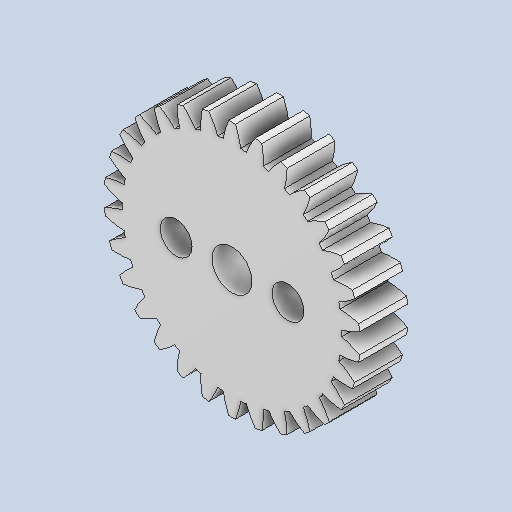
# Autodesk Inventor part: 平歯車1
Saved by Autodesk Inventor 2025.2 (Build 292293000, 293)
## iProperties
CustomPartVersion: 1
Created: 2024-12-16
Part Number: 平歯車1
Material: ABS プラスチック
Document SubType Name: Modeling
Designer: haruy
Categories: <?xml version="1.0" encoding="UTF-16"?> <MemberInstance><Categories><FamilyTemplate><FamilyTemplateParameter ValueType="xs:double" Id="1" ObjectReferenceKey="da_z" ObjectType="kUserParameterObject"/><FamilyTemplateParameter ValueType="xs:double" Id="2" ObjectReferenceKey="da_b" ObjectType="kUserParameterObject"/><FamilyTemplateParameter ValueType="xs:double" Id="3" ObjectReferenceKey="da_beta" ObjectType="kUserParameterObject"/><FamilyTemplateParameter ValueType="xs:double" Id="4" ObjectReferenceKey="da_da" ObjectType="kUserParameterObject"/><FamilyTemplateParameter ValueType="xs:double" Id="5" ObjectReferenceKey="da_aw" ObjectType="kUserParameterObject"/><FamilyTemplateParameter ValueType="xs:string" Id="6" ObjectReferenceKey="EAIAABAAAACIAQAAAAAAAIAAAAAAAAAA" ObjectType="83910656" SubObjectId="SurfaceGeometry"/></FamilyTemplate><ParamToTemplateMap><ParamToTemplate CategoryParameter="//CategoryParameter[@InternalName='046C89C9-8512-4d59-83FE-43B91F4F132A']" TemplateParameter="1"/><ParamToTemplate CategoryParameter="//CategoryParameter[@InternalName='2552DF32-E462-4b46-AEBF-C6C7768E72AC']" TemplateParameter="2"/><ParamToTemplate CategoryParameter="//CategoryParameter[@InternalName='C9EE641D-15FC-4fae-A226-E94C4372FDD7']" TemplateParameter="3"/><ParamToTemplate><ParamToTemplate CategoryParameter="//CategoryParameter[@InternalName='00B6519A-459B-49c7-AD84-2E56D39A5744']" ConstantValue="0.000000"/></ParamToTemplate><ParamToTemplate><ParamToTemplate CategoryParameter="//CategoryParameter[@InternalName='04B31F0E-C7A6-4894-AA32-9629BEFACF47']" ConstantValue="1.000000"/></ParamToTemplate><ParamToTemplate><ParamToTemplate CategoryParameter="//CategoryParameter[@InternalName='43CBEC2E-7847-49e7-A936-2F7889FCB2D9']" ConstantValue="0.250000"/></ParamToTemplate><ParamToTemplate><ParamToTemplate CategoryParameter="//CategoryParameter[@InternalName='B1EFC894-105D-4ebd-86BF-FA20ED196853']" ConstantValue="0.350000"/></ParamToTemplate><ParamToTemplate><ParamToTemplate CategoryParameter="//CategoryParameter[@InternalName='51175063-3D10-4879-93E8-6246FE8B403D']" ConstantValue="2060000000.000000"/></ParamToTemplate><ParamToTemplate><ParamToTemplate CategoryParameter="//CategoryParameter[@InternalName='A3A52E27-4454-46a9-B0BD-C932399B70AF']" ConstantValue="0.300000"/></ParamToTemplate><ParamToTemplate><ParamToTemplate CategoryParameter="//CategoryParameter[@InternalName='91B76062-C214-41d9-B1B9-14D2AB99603D']" ConstantValue="0.100000"/></ParamToTemplate><ParamToTemplate><ParamToTemplate CategoryParameter="//CategoryParameter[@InternalName='374E806E-8B8A-4dda-A9AA-1039D6500AD2']" ConstantValue="10.000000"/></ParamToTemplate><ParamToTemplate><ParamToTemplate CategoryParameter="//CategoryParameter[@InternalName='2D373A89-B862-43d6-8D0B-0CBF12AB9F6C']" ConstantValue="0.349066"/></ParamToTemplate><ParamToTemplate CategoryParameter="//CategoryParameter[@InternalName='37777632-D6A2-4fac-9D53-DB8ACD95C989']" TemplateParameter="4"/><ParamToTemplate CategoryParameter="//CategoryParameter[@InternalName='FD1017F1-B727-4f7e-9707-0F86F1FF9423']" TemplateParameter="5"/><ParamToTemplate><ParamToTemplate CategoryParameter="//CategoryParameter[@InternalName='9E1B4470-B2D3-4ff1-B813-535BB4CDF51A']" ConstantValue="3520000.000000"/></ParamToTemplate><ParamToTemplate><ParamToTemplate CategoryParameter="//CategoryParameter[@InternalName='F8452263-BFF6-458c-9FB1-07C4B99E95CD']" ConstantValue="11400000.000000"/></ParamToTemplate><ParamToTemplate><ParamToTemplate CategoryParameter="//CategoryParameter[@InternalName='3E3BB259-FD49-497f-8171-6EBC954A3479']" ConstantValue="2.000000"/></ParamToTemplate><ParamToTemplate CategoryParameter="//CategoryParameter[@InternalName='27C3BAF2-7550-4e4b-AE2C-0DB134B7D9B7']" TemplateParameter="6"/></ParamToTemplateMap><Category DisplayName="Gear" InternalName="DC85795E-93AB-48d5-8EEE-5A27447B64BD" Mnemonic="Gear"><CategoryParameter DisplayName="z" InternalName="046C89C9-8512-4d59-83FE-43B91F4F132A" Mnemonic="z"/><CategoryParameter DisplayName="b" InternalName="2552DF32-E462-4b46-AEBF-C6C7768E72AC" Mnemonic="b"/><CategoryParameter DisplayName="||b|" InternalName="C9EE641D-15FC-4fae-A226-E94C4372FDD7" Mnemonic="beta"/><CategoryParameter DisplayName="x" InternalName="00B6519A-459B-49c7-AD84-2E56D39A5744" Mnemonic="x"/><CategoryParameter DisplayName="a*" InternalName="04B31F0E-C7A6-4894-AA32-9629BEFACF47" Mnemonic="a"/><CategoryParameter DisplayName="c*" InternalName="43CBEC2E-7847-49e7-A936-2F7889FCB2D9" Mnemonic="c"/><CategoryParameter DisplayName="r|.f|*" InternalName="B1EFC894-105D-4ebd-86BF-FA20ED196853" Mnemonic="rf"/><CategoryParameter DisplayName="E" InternalName="51175063-3D10-4879-93E8-6246FE8B403D" Mnemonic="E"/><CategoryParameter DisplayName="||m|" InternalName="A3A52E27-4454-46a9-B0BD-C932399B70AF" Mnemonic="mi"/><Category DisplayName="SpurGear" InternalName="26C5A22E-A91E-4dfd-A3B3-23CCAFAE1764" Mnemonic="SpurGear"><CategoryParameter DisplayName="m" InternalName="91B76062-C214-41d9-B1B9-14D2AB99603D" Mnemonic="m"/><CategoryParameter DisplayName="P" InternalName="374E806E-8B8A-4dda-A9AA-1039D6500AD2" Mnemonic="PP"/><CategoryParameter DisplayName="||a|" InternalName="2D373A89-B862-43d6-8D0B-0CBF12AB9F6C" Mnemonic="alpha"/><CategoryParameter DisplayName="d|.a|" InternalName="37777632-D6A2-4fac-9D53-DB8ACD95C989" Mnemonic="da"/><CategoryParameter DisplayName="a|.w|" InternalName="FD1017F1-B727-4f7e-9707-0F86F1FF9423" Mnemonic="aw"/><CategoryParameter DisplayName="||s||.Flim|" InternalName="9E1B4470-B2D3-4ff1-B813-535BB4CDF51A" Mnemonic="sFlim"/><CategoryParameter DisplayName="||s||.Hlim|" InternalName="F8452263-BFF6-458c-9FB1-07C4B99E95CD" Mnemonic="sHlim"/><CategoryParameter DisplayName="タイプ" InternalName="3E3BB259-FD49-497f-8171-6EBC954A3479" Mnemonic="type"/><CategoryParameter DisplayName="PitchDiameter" InternalName="27C3BAF2-7550-4e4b-AE2C-0DB134B7D9B7" Mnemonic="IDS_PITCHDIAM"/></Category></Category></Categories></MemberInstance>
Density: 1.06 g/cm^3
Appearance: 滑らか - 白
Author: haruy
Autodesk Inventor part; units mm, degrees
sketch "Sketch1" plane through (0, 0, 0) normal (0, 0, 1) x (1, 0, 0)
  circle A0 centre (0, 0) radius 16
  dimension "d0" = 32
  constraints: 1 centre point
  measures "d0" diameter of A0
extrude "Extrusion1" add sketch "Sketch1" along normal blind 6
ref_plane "Work Plane2" through (0, 0, 3) normal (0, 0, 1) x (1, 0, 0)
sketch "Sketch2" plane through (0, 0, 0) normal (0, 0, -1) x (-1, 0, 0)
  circle A0 centre (0, 0) radius 16 projected
  circle A1 centre (0, 0) radius 15
  dimension "d3" = 30
  constraints: 1 centre point, 1 coincident
  measures "d3" diameter of A1
surface extrude "ピッチ円直径" sketch "Sketch2" against normal through all shown no curves A1
ref_plane "Work Plane8" through (0, 0, 0) normal (0.9945219, 0.1045285, 0) x (0, 0, 1)
ref_plane "Work Plane9" through (0, 0, 0) normal (1, 0, 0) x (0, 1, 0)
spur gear teeth "平歯車" teeth 30 pitch diameter 30 tip diameter 32 root diameter 27.5 face width 6 start plane through (0, 0, 0) normal (0, 0, -1) x (-1, 0, 0)
sketch "スケッチ3" plane through (0, 0, 6) normal (0, 0, 1) x (1, 0, 0)
  circle A0 centre (0, 0) radius 2.5
  circle A1 centre (-7, 0) radius 2
  circle A2 centre (7, 0) radius 2
  dimension "d49" = 5
  dimension "d50" = 4
  dimension "d52" = 7
  dimension "d54" = 0
  dimension "d57" = 360
  constraints: 3 centre point, 1 coincident, 5 other
  measures "d49" diameter of A0
  measures "d50" diameter of A1
  measures "d52" distance of A1.centre point (0, 0)
  measures "d54" vertical distance of A1.centre point (0, 0)
extrude "押し出し2" cut sketch "スケッチ3" against normal blind 10
sketch "スケッチ4" plane through (0, 0, 6) normal (0, 0, 1) x (1, 0, 0)
  circle A0 centre (-7, 0) radius 2 projected
  circle A1 centre (7, 0) radius 2 projected
  circle A2 centre (0, 0) radius 2.5 projected
  arc A3 (-3.7351, 15.5579) -> (-3.9052, 13.1838) centre (6.0885, 13.661) ccw projected
  arc A4 (-3.9052, 13.1838) -> (-4.5898, 12.9613) centre (0, 0) ccw projected
  arc A5 (-4.5898, 12.9613) -> (-6.1229, 14.7821) centre (-12.9554, 7.4732) ccw projected
  arc A6 (-6.1229, 14.7821) -> (-6.8882, 14.4414) centre (0, 0) ccw projected
  arc A7 (-6.8882, 14.4414) -> (-6.5609, 12.0837) centre (3.1152, 14.6283) ccw projected
  arc A8 (-6.5609, 12.0837) -> (-7.1844, 11.7238) centre (0, 0) ccw projected
  arc A9 (-7.1844, 11.7238) -> (-9.0625, 13.186) centre (-14.2261, 4.6164) ccw projected
  arc A10 (-9.0625, 13.186) -> (-9.7402, 12.6937) centre (0, 0) ccw projected
  arc A11 (-9.7402, 12.6937) -> (-8.9299, 10.4556) centre (0.0057, 14.9563) ccw projected
  arc A12 (-8.9299, 10.4556) -> (-9.4649, 9.9739) centre (0, 0) ccw projected
  arc A13 (-9.4649, 9.9739) -> (-11.606, 11.0137) centre (-14.875, 1.5577) ccw projected
  arc A14 (-11.606, 11.0137) -> (-12.1665, 10.3912) centre (0, 0) ccw projected
  arc A15 (-12.1665, 10.3912) -> (-10.9086, 8.3705) centre (-3.104, 14.6307) ccw projected
  arc A16 (-10.9086, 8.3705) -> (-11.3317, 7.7881) centre (0, 0) ccw projected
  arc A17 (-11.3317, 7.7881) -> (-13.6422, 8.36) centre (-14.8738, -1.569) ccw projected
  arc A18 (-13.6422, 8.36) -> (-14.0611, 7.6345) centre (0, 0) ccw projected
  arc A19 (-14.0611, 7.6345) -> (-12.4105, 5.9195) centre (-6.0781, 13.6656) ccw projected
  arc A20 (-12.4105, 5.9195) -> (-12.7033, 5.2619) centre (0, 0) ccw projected
  arc A21 (-12.7033, 5.2619) -> (-15.0823, 5.3409) centre (-14.2226, -4.6272) ccw projected
  arc A22 (-15.0823, 5.3409) -> (-15.3411, 4.5442) centre (0, 0) ccw projected
  arc A23 (-15.3411, 4.5442) -> (-13.3701, 3.2099) centre (-8.7865, 12.1033) ccw projected
  arc A24 (-13.3701, 3.2099) -> (-13.5198, 2.5057) centre (0, 0) ccw projected
  arc A25 (-13.5198, 2.5057) -> (-15.8631, 2.0884) centre (-12.9497, -7.4831) ccw projected
  arc A26 (-15.8631, 2.0884) -> (-15.9507, 1.2553) centre (0, 0) ccw projected
  arc A27 (-15.9507, 1.2553) -> (-13.7453, 0.3599) centre (-11.1109, 10.012) ccw projected
  arc A28 (-13.7453, 0.3599) -> (-13.7453, -0.3599) centre (0, 0) ccw projected
  arc A29 (-13.7453, -0.3599) -> (-15.9507, -1.2553) centre (-11.1109, -10.012) ccw projected
  arc A30 (-15.9507, -1.2553) -> (-15.8631, -2.0884) centre (0, 0) ccw projected
  arc A31 (-15.8631, -2.0884) -> (-13.5198, -2.5057) centre (-12.9497, 7.4831) ccw projected
  arc A32 (-13.5198, -2.5057) -> (-13.3701, -3.2099) centre (0, 0) ccw projected
  arc A33 (-13.3701, -3.2099) -> (-15.3411, -4.5442) centre (-8.7865, -12.1033) ccw projected
  arc A34 (-15.3411, -4.5442) -> (-15.0823, -5.3409) centre (0, 0) ccw projected
  arc A35 (-15.0823, -5.3409) -> (-12.7033, -5.2619) centre (-14.2226, 4.6272) ccw projected
  arc A36 (-12.7033, -5.2619) -> (-12.4105, -5.9195) centre (0, 0) ccw projected
  arc A37 (-12.4105, -5.9195) -> (-14.0611, -7.6345) centre (-6.0781, -13.6656) ccw projected
  arc A38 (-14.0611, -7.6345) -> (-13.6422, -8.36) centre (0, 0) ccw projected
  arc A39 (-13.6422, -8.36) -> (-11.3317, -7.7881) centre (-14.8738, 1.569) ccw projected
  arc A40 (-11.3317, -7.7881) -> (-10.9086, -8.3705) centre (0, 0) ccw projected
  arc A41 (-10.9086, -8.3705) -> (-12.1665, -10.3912) centre (-3.104, -14.6307) ccw projected
  arc A42 (-12.1665, -10.3912) -> (-11.606, -11.0137) centre (0, 0) ccw projected
  arc A43 (-11.606, -11.0137) -> (-9.4649, -9.9739) centre (-14.875, -1.5577) ccw projected
  arc A44 (-9.4649, -9.9739) -> (-8.9299, -10.4556) centre (0, 0) ccw projected
  arc A45 (-8.9299, -10.4556) -> (-9.7402, -12.6937) centre (0.0057, -14.9563) ccw projected
  arc A46 (-9.7402, -12.6937) -> (-9.0625, -13.186) centre (0, 0) ccw projected
  arc A47 (-9.0625, -13.186) -> (-7.1844, -11.7238) centre (-14.2261, -4.6164) ccw projected
  arc A48 (-7.1844, -11.7238) -> (-6.5609, -12.0837) centre (0, 0) ccw projected
  arc A49 (-6.5609, -12.0837) -> (-6.8882, -14.4414) centre (3.1152, -14.6283) ccw projected
  arc A50 (-6.8882, -14.4414) -> (-6.1229, -14.7821) centre (0, 0) ccw projected
  arc A51 (-6.1229, -14.7821) -> (-4.5898, -12.9613) centre (-12.9554, -7.4732) ccw projected
  arc A52 (-4.5898, -12.9613) -> (-3.9052, -13.1838) centre (0, 0) ccw projected
  arc A53 (-3.9052, -13.1838) -> (-3.7351, -15.5579) centre (6.0885, -13.661) ccw projected
  arc A54 (-3.7351, -15.5579) -> (-2.9158, -15.7321) centre (0, 0) ccw projected
  arc A55 (-2.9158, -15.7321) -> (-1.7947, -13.6324) centre (-11.1185, -10.0035) ccw projected
  arc A56 (-1.7947, -13.6324) -> (-1.0788, -13.7076) centre (0, 0) ccw projected
  arc A57 (-1.0788, -13.7076) -> (-0.4188, -15.9945) centre (8.7957, -12.0966) ccw projected
  arc A58 (-0.4188, -15.9945) -> (0.4188, -15.9945) centre (0, 0) ccw projected
  arc A59 (0.4188, -15.9945) -> (1.0788, -13.7076) centre (-8.7957, -12.0966) ccw projected
  arc A60 (1.0788, -13.7076) -> (1.7947, -13.6324) centre (0, 0) ccw projected
  arc A61 (1.7947, -13.6324) -> (2.9158, -15.7321) centre (11.1185, -10.0035) ccw projected
  arc A62 (2.9158, -15.7321) -> (3.7351, -15.5579) centre (0, 0) ccw projected
  arc A63 (3.7351, -15.5579) -> (3.9052, -13.1838) centre (-6.0885, -13.661) ccw projected
  arc A64 (3.9052, -13.1838) -> (4.5898, -12.9613) centre (0, 0) ccw projected
  arc A65 (4.5898, -12.9613) -> (6.1229, -14.7821) centre (12.9554, -7.4732) ccw projected
  arc A66 (6.1229, -14.7821) -> (6.8882, -14.4414) centre (0, 0) ccw projected
  arc A67 (6.8882, -14.4414) -> (6.5609, -12.0837) centre (-3.1152, -14.6283) ccw projected
  arc A68 (6.5609, -12.0837) -> (7.1844, -11.7238) centre (0, 0) ccw projected
  arc A69 (7.1844, -11.7238) -> (9.0625, -13.186) centre (14.2261, -4.6164) ccw projected
  arc A70 (9.0625, -13.186) -> (9.7402, -12.6937) centre (0, 0) ccw projected
  arc A71 (9.7402, -12.6937) -> (8.9299, -10.4556) centre (-0.0057, -14.9563) ccw projected
  arc A72 (8.9299, -10.4556) -> (9.4649, -9.9739) centre (0, 0) ccw projected
  arc A73 (9.4649, -9.9739) -> (11.606, -11.0137) centre (14.875, -1.5577) ccw projected
  arc A74 (11.606, -11.0137) -> (12.1665, -10.3912) centre (0, 0) ccw projected
  arc A75 (12.1665, -10.3912) -> (10.9086, -8.3705) centre (3.104, -14.6307) ccw projected
  arc A76 (10.9086, -8.3705) -> (11.3317, -7.7881) centre (0, 0) ccw projected
  arc A77 (11.3317, -7.7881) -> (13.6422, -8.36) centre (14.8738, 1.569) ccw projected
  arc A78 (13.6422, -8.36) -> (14.0611, -7.6345) centre (0, 0) ccw projected
  arc A79 (14.0611, -7.6345) -> (12.4105, -5.9195) centre (6.0781, -13.6656) ccw projected
  arc A80 (12.4105, -5.9195) -> (12.7033, -5.2619) centre (0, 0) ccw projected
  arc A81 (12.7033, -5.2619) -> (15.0823, -5.3409) centre (14.2226, 4.6272) ccw projected
  arc A82 (15.0823, -5.3409) -> (15.3411, -4.5442) centre (0, 0) ccw projected
  arc A83 (15.3411, -4.5442) -> (13.3701, -3.2099) centre (8.7865, -12.1033) ccw projected
  arc A84 (13.3701, -3.2099) -> (13.5198, -2.5057) centre (0, 0) ccw projected
  arc A85 (13.5198, -2.5057) -> (15.8631, -2.0884) centre (12.9497, 7.4831) ccw projected
  arc A86 (15.8631, -2.0884) -> (15.9507, -1.2553) centre (0, 0) ccw projected
  arc A87 (15.9507, -1.2553) -> (13.7453, -0.3599) centre (11.1109, -10.012) ccw projected
  arc A88 (13.7453, -0.3599) -> (13.7453, 0.3599) centre (0, 0) ccw projected
  arc A89 (13.7453, 0.3599) -> (15.9507, 1.2553) centre (11.1109, 10.012) ccw projected
  arc A90 (15.9507, 1.2553) -> (15.8631, 2.0884) centre (0, 0) ccw projected
  arc A91 (15.8631, 2.0884) -> (13.5198, 2.5057) centre (12.9497, -7.4831) ccw projected
  arc A92 (13.5198, 2.5057) -> (13.3701, 3.2099) centre (0, 0) ccw projected
  arc A93 (13.3701, 3.2099) -> (15.3411, 4.5442) centre (8.7865, 12.1033) ccw projected
  arc A94 (15.3411, 4.5442) -> (15.0823, 5.3409) centre (0, 0) ccw projected
  arc A95 (15.0823, 5.3409) -> (12.7033, 5.2619) centre (14.2226, -4.6272) ccw projected
  arc A96 (12.7033, 5.2619) -> (12.4105, 5.9195) centre (0, 0) ccw projected
  arc A97 (12.4105, 5.9195) -> (14.0611, 7.6345) centre (6.0781, 13.6656) ccw projected
  arc A98 (14.0611, 7.6345) -> (13.6422, 8.36) centre (0, 0) ccw projected
  arc A99 (13.6422, 8.36) -> (11.3317, 7.7881) centre (14.8738, -1.569) ccw projected
  arc A100 (11.3317, 7.7881) -> (10.9086, 8.3705) centre (0, 0) ccw projected
  arc A101 (10.9086, 8.3705) -> (12.1665, 10.3912) centre (3.104, 14.6307) ccw projected
  arc A102 (12.1665, 10.3912) -> (11.606, 11.0137) centre (0, 0) ccw projected
  arc A103 (11.606, 11.0137) -> (9.4649, 9.9739) centre (14.875, 1.5577) ccw projected
  arc A104 (9.4649, 9.9739) -> (8.9299, 10.4556) centre (0, 0) ccw projected
  arc A105 (8.9299, 10.4556) -> (9.7402, 12.6937) centre (-0.0057, 14.9563) ccw projected
  arc A106 (9.7402, 12.6937) -> (9.0625, 13.186) centre (0, 0) ccw projected
  arc A107 (9.0625, 13.186) -> (7.1844, 11.7238) centre (14.2261, 4.6164) ccw projected
  arc A108 (7.1844, 11.7238) -> (6.5609, 12.0837) centre (0, 0) ccw projected
  arc A109 (6.5609, 12.0837) -> (6.8882, 14.4414) centre (-3.1152, 14.6283) ccw projected
  arc A110 (6.8882, 14.4414) -> (6.1229, 14.7821) centre (0, 0) ccw projected
  arc A111 (6.1229, 14.7821) -> (4.5898, 12.9613) centre (12.9554, 7.4732) ccw projected
  arc A112 (4.5898, 12.9613) -> (3.9052, 13.1838) centre (0, 0) ccw projected
  arc A113 (3.9052, 13.1838) -> (3.7351, 15.5579) centre (-6.0885, 13.661) ccw projected
  arc A114 (3.7351, 15.5579) -> (2.9158, 15.7321) centre (0, 0) ccw projected
  arc A115 (2.9158, 15.7321) -> (1.7947, 13.6324) centre (11.1185, 10.0035) ccw projected
  arc A116 (1.7947, 13.6324) -> (1.0788, 13.7076) centre (0, 0) ccw projected
  arc A117 (1.0788, 13.7076) -> (0.4188, 15.9945) centre (-8.7957, 12.0966) ccw projected
  arc A118 (0.4188, 15.9945) -> (-0.4188, 15.9945) centre (0, 0) ccw projected
  arc A119 (-0.4188, 15.9945) -> (-1.0788, 13.7076) centre (8.7957, 12.0966) ccw projected
  arc A120 (-1.0788, 13.7076) -> (-1.7947, 13.6324) centre (0, 0) ccw projected
  arc A121 (-1.7947, 13.6324) -> (-2.9158, 15.7321) centre (-11.1185, 10.0035) ccw projected
  arc A122 (-2.9158, 15.7321) -> (-3.7351, 15.5579) centre (0, 0) ccw projected
equation "\"d0\" = da_da"
equation "\"d1\" = da_b"
equation "\"d3\" = da_d"
equation "\"da_da\" = 32"
equation "\"da_b\" = 6"
equation "\"da_d\" = 30"
body "Solid1"
body "Srf1"
